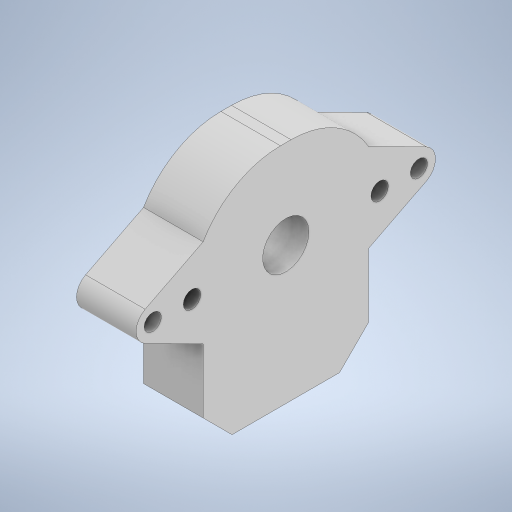
# Autodesk Inventor part: AMT102-0512-I5000-5
Saved by Autodesk Inventor 2024 (Build 280153000, 153)
## iProperties
Created: 2025-12-10
Part Number: AMT102-0512-I5000-5
Material: Generic
Document SubType Name: Modeling
Designer: schar
Density: 1 g/cm^3
Appearance: Default
Author: schar
Autodesk Inventor part; units mm, degrees
ref_plane "YZ Plane" through (0, 0, 0) normal (1, 0, 0) x (0, 1, 0)
ref_plane "XZ Plane" through (0, 0, 0) normal (0, 1, 0) x (-1, 0, 0)
ref_plane "XY Plane" through (0, 0, 0) normal (0, 0, 1) x (1, 0, 0)
sketch "Sketch1" plane through (0, 0, 0) normal (1, 0, 0) x (0, 1, 0)
  line L0 (-0.54, 0) -> (-0.54, -14.29)
  circle A0 centre (-0.54, 0) radius 7.65
  line L1 (-0.54, -14.29) -> (14.79, -14.29)
  line L2 (14.79, -14.29) -> (-24.27, -14.29)
  line L3 (-24.27, -14.29) -> (-24.27, 14.29)
  line L4 (-24.27, 14.29) -> (14.79, 14.29)
  line L5 (14.79, 14.29) -> (14.79, -14.29)
  circle A1 centre (-0.54, 0) radius 16.22
  circle A2 centre (-0.54, 0) radius 23.01
  line L6 (-0.54, 0) -> (-0.54, -23.01)
  line L7 (-0.54, -23.01) -> (-0.54, -24.49)
  line L8 (-0.54, -23.01) -> (0.895, -23.01)
  ellipse E0 centre (-0.54, -23.01) end of major axis (-0.54, -24.49) minor radius 1.435
  circle A3 centre (-0.54, -16.22) radius 1.5
  line L9 (-8.19, 0) -> (-16.76, 0)
  line L10 (-8.19, 0) -> (-8.19, -14.29)
  line L11 (-0.54, -23.01) -> (-3.41, -23.01)
  circle A4 centre (-0.54, -23.01) radius 2.87
  line L12 (-8.19, -14.29) -> (-3.0986, -24.3101)
  line L13 (7.11, -14.29) -> (2.0186, -24.3101)
  ellipse E1 centre (-0.54, 23.01) end of major axis (-0.54, 24.49) minor radius 1.435
  circle A5 centre (-0.54, 16.22) radius 1.5
  circle A6 centre (-0.54, 23.01) radius 2.87
  line L14 (-8.19, 14.29) -> (-3.0986, 24.3101)
  line L15 (7.11, 14.29) -> (2.0186, 24.3101)
  point P0 (-3.4044, -22.831)
  point P1 (-1.9743, -22.9653)
  point P2 (-1.975, -23.01)
  point P3 (-8.1812, -14.3074)
  point P4 (-8.1812, 14.3074)
  point P5 (-8.2136, 14.29)
  point P6 (-8.2136, -14.29)
  dimension "d13" = 15.3
  dimension "d18" = 46.02
  dimension "d12" = 14.29
  dimension "d14" = 15.33
  dimension "d15" = 39.06
  dimension "d16" = 28.58
  dimension "d17" = 32.44
  dimension "d19" = 1.48
  dimension "d20" = 1.435
  dimension "d21" = 3
  dimension "d22" = 2.87
  constraints: 32 end point, 9 symmetric about line, 6 coincident, 6 horizontal, 4 centre point, 4 point on circle, 4 vertical, 2 parallel, 2 perpendicular, 2 point on line, 1 horizontal alignment, 1 tangent, 16 other
  measures "d12" distance of L0.start L0.end
  measures "d14" distance of L0.end L1.end
  measures "d15" distance of L3.end L4.end
  measures "d16" distance of L2.end L3.end
  measures "d17" diameter of A1
  measures "d19" distance of L6.end L7.end
  measures "d20" distance of L6.end L8.end
  measures "d21" diameter of A3
  measures "d22" distance of L11.start L11.end
extrude "Extrusion1" add sketch "Sketch1" along normal blind 10.3 contours A0 L9 A1 L4 L5 L1 L0 | L0 L2 L10 A0 | L6 A3 A1 L12 L2 | L1 L13 A1 A3 L6 | L10 L2 A1 L9 | L12 A1 L2 | A1 L2 A2 L4 | A1 L5 L1 | L13 A2 A4 L6 A3 A1 | A1 A3 L6 A4 A2 L12 | A1 L14 L4 | L13 A4 A2 | L2 L3 L4 A2 | A2 A4 L12 | L14 A1 A5 L15 L4 | L14 A2 A6 L15 A1 A5 | A1 L4 L5 | A4 L11 E0 A2 | A2 E0 L6 A4 | A4 L6 E0 A2 | A2 E0 L11 A4 | L14 A6 A2 | A2 A6 L15 | A6 A2 E1 | A2 E1 A6
fillet "Fillet1" radius 15.49 2 edges at (5.15, 14.79, -14.29) (5.15, 14.79, 14.29)
chamfer "Chamfer1" distance 5 angle 45 2 edges at (5.15, -24.27, -14.29) (5.15, -24.27, 14.29)
sketch "Sketch2" plane through (10.3, 0, 0) normal (1, 0, 0) x (0, 0, -1)
  circle A0 centre (0, -0.54) radius 7.65 projected
  line L0 (0, -0.54) -> (7.65, -0.54)
  circle A1 centre (0, -0.54) radius 4
  circle A2 centre (0, -0.54) radius 7.65
  point P0 (0, 0)
  dimension "d29" = 8
  constraints: 2 coincident, 2 end point, 2 horizontal alignment, 1 centre point, 1 horizontal, 3 other
  measures "d29" diameter of A1
extrude "8mm_inlet" add sketch "Sketch2" against normal up to surface (10.3 mm away)
body "Solid1"
